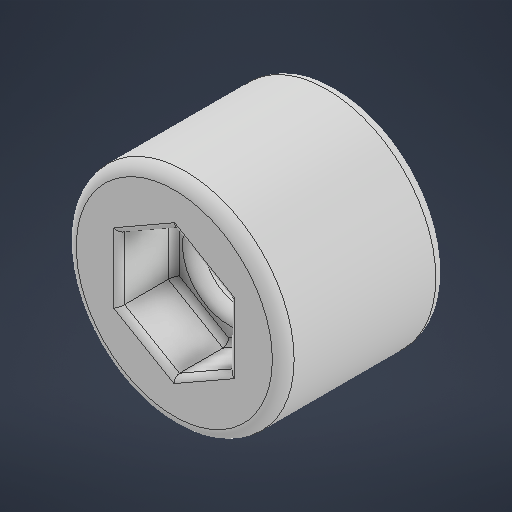
# Autodesk Inventor part: ExtensionFastener
Saved by Autodesk Inventor 2026.2 (Build 302298010, 298A)
## iProperties
Created: 2026-06-23
Part Number: ExtensionFastener
Material: Generic
Document SubType Name: Modeling
Designer: frede
Density: 1 g/cm^3
Appearance: Default
Author: frede
Autodesk Inventor part; units mm, degrees
ref_plane "YZ Plane" through (0, 0, 0) normal (1, 0, 0) x (0, 1, 0)
ref_plane "XZ Plane" through (0, 0, 0) normal (0, 1, 0) x (-1, 0, 0)
ref_plane "XY Plane" through (0, 0, 0) normal (0, 0, 1) x (1, 0, 0)
sketch "Sketch2" plane through (0, 0, 0) normal (0, 0, 1) x (1, 0, 0)
  circle A0 centre (0, 0) radius 10
  circle A1 centre (0, 0) radius 3.25
  dimension "d0" = 20
  dimension "d1" = 6.5
  constraints: 2 centre point, 2 coincident
  measures "d0" diameter of A0
  measures "d1" diameter of A1
extrude "Extrusion1" add sketch "Sketch2" along normal blind 15
sketch "Sketch3" plane through (0, 0, 15) normal (0, 0, 1) x (1, 0, 0)
  circle A0 centre (0, 0) radius 3.25 projected
  line L0 (5.0629, 2.8931) -> (5.037, -2.9381)
  line L1 (5.037, -2.9381) -> (-0.026, -5.8312)
  line L2 (-0.026, -5.8312) -> (-5.0629, -2.8931)
  line L3 (-5.0629, -2.8931) -> (-5.037, 2.9381)
  line L4 (-5.037, 2.9381) -> (0.026, 5.8312)
  line L5 (0.026, 5.8312) -> (5.0629, 2.8931)
  dimension "d4" = 10.1
  constraints: 12 end point, 1 coincident, 13 other
  measures "d4" distance between parallel lines of L0 L3
extrude "Extrusion2" cut sketch "Sketch3" against normal blind 5
fillet "Fillet1" radius 0.5 12 edges at (-2.5055, 4.3846, 15) (2.5444, 4.3621, 15) (5.0499, -0.0225, 15) (2.5055, -4.3846, 15) (-2.5444, -4.3621, 15) (-5.0499, 0.0225, 15) (-5.0499, 0.0225, 10) (-2.5055, 4.3846, 10) (2.5444, 4.3621, 10) (5.0499, -0.0225, 10) (2.5055, -4.3846, 10) (-2.5444, -4.3621, 10)
fillet "Fillet2" radius 1 4 edges at (-3.25, 0, 10) (-3.25, 0, 0) (-10, 0, 15) (-10, 0, 0)
body "Solid1"
